Battery Top Spacer_v2 (Autodesk Fusion 360 design; units mm, degrees)
Autodesk Fusion 360 part; units mm, degrees
sketch "Sketch1" plane through (0, 0, 0) normal (1, 0, 0) x (0, 1, 0)
  line L0 (7.1607, -3.9) -> (12.8393, -3.9)
  line L1 (4.5, -8.2) -> (4.5, -6.5607)
  line L2 (12.8393, 3.9) -> (7.1607, 3.9)
  arc A0 (6.8786, -8.5414) -> (6.7372, -8.2) centre (6.7372, -8.4) ccw
  circle A1 centre (10, 0) radius 2.1
  arc A2 (5.1, -10) -> (5.5978, -9.8222) centre (5.1591, -9.3798) ccw
  line L3 (12.8393, 3.9) -> (7.1607, 3.9)
  line L4 (6.1, 2.8393) -> (6.1, -2.8393)
  line L5 (6.7372, -8.2) -> (4.5, -8.2)
  line L6 (6.1, 2.8393) -> (6.1, -2.8393)
  line L7 (4.5, -6.5607) -> (7.1607, -3.9)
  line L8 (5.5978, -9.8222) -> (6.8786, -8.5414)
  arc A3 (5.1, -10) -> (5.5978, -9.8222) centre (5.1591, -9.3798) ccw
  arc A4 (6.8786, -8.5414) -> (6.7372, -8.2) centre (6.7372, -8.4) ccw
  line L9 (6.7372, -8.2) -> (4.5, -8.2)
  line L10 (4.5, -8.2) -> (4.5, -6.5607)
  line L11 (4.5, -6.5607) -> (7.1607, -3.9)
  line L12 (5.5978, -9.8222) -> (6.8786, -8.5414)
  line L13 (7.1607, -3.9) -> (12.8393, -3.9)
  arc A5 (14.4022, -9.8222) -> (14.9, -10) centre (14.8416, -9.3778) ccw
  line L14 (26.7372, -8.2) -> (24.5, -8.2)
  line L15 (-18.2, 3.2628) -> (-18.2, 5.5)
  line L16 (33.2628, 8.2) -> (35.5, 8.2)
  line L17 (-18.2, 3.2628) -> (-18.2, 5.5)
  line L18 (24.5, -6.5607) -> (27.1607, -3.9)
  arc A6 (-14.8314, -10) -> (-14.4022, -9.8222) centre (-14.8314, -9.3929) ccw
  arc A7 (26.8786, -8.5414) -> (26.7372, -8.2) centre (26.7372, -8.4) ccw
  line L19 (38.2, 5.5) -> (38.2, 3.2628)
  arc A8 (38.2, 3.2628) -> (38.5414, 3.1214) centre (38.4, 3.2628) ccw
  line L20 (13.1214, -8.5414) -> (14.4022, -9.8222)
  arc A9 (40, 9.5) -> (39.5, 10) centre (39.5, 9.5) ccw
  arc A10 (-13.1214, -8.5414) -> (-13.2628, -8.2) centre (-13.2628, -8.4) ccw
  line L21 (22.7, -8.2) -> (17.3, -8.2)
  line L22 (36.5607, -5.5) -> (33.9, -2.8393)
  line L23 (-20, -4.8314) -> (-20, -9.5)
  line L24 (36.5607, 5.5) -> (38.2, 5.5)
  arc A11 (-18.2, -3.2628) -> (-18.5414, -3.1214) centre (-18.4, -3.2628) ccw
  arc A12 (39.5, -10) -> (40, -9.5) centre (39.5, -9.5) ccw
  arc A13 (33.1214, 8.5414) -> (33.2628, 8.2) centre (33.2628, 8.4) ccw
  line L25 (33.2628, 8.2) -> (35.5, 8.2)
  arc A14 (-14.8314, -10) -> (-14.4022, -9.8222) centre (-14.8314, -9.3929) ccw
  line L26 (40, -9.5) -> (40, -4.8314)
  line L27 (-13.2628, -8.2) -> (-15.5, -8.2)
  line L28 (38.2, 5.5) -> (38.2, 3.2628)
  line L29 (-13.2628, -8.2) -> (-15.5, -8.2)
  line L30 (33.9, 2.8393) -> (36.5607, 5.5)
  line L31 (33.1214, -8.5414) -> (34.4022, -9.8222)
  line L32 (-18.2, 5.5) -> (-16.5607, 5.5)
  line L33 (39.8222, -4.4022) -> (38.5414, -3.1214)
  arc A15 (34.4022, -9.8222) -> (34.8314, -10) centre (34.8314, -9.3929) ccw
  arc A16 (38.5414, -3.1214) -> (38.2, -3.2628) centre (38.4, -3.2628) ccw
  line L34 (35.5, -8.2) -> (33.2628, -8.2)
  line L35 (15.5, -6.5607) -> (15.5, -8.2)
  line L36 (-14.9, 10) -> (-19.5, 10)
  line L37 (32.8393, -3.9) -> (35.5, -6.5607)
  arc A17 (25.1, -10) -> (25.5978, -9.8222) centre (25.1584, -9.3778) ccw
  line L38 (24.5, -6.5607) -> (27.1607, -3.9)
  line L39 (15.5, -6.5607) -> (15.5, -8.2)
  line L40 (39.8222, -4.4022) -> (38.5414, -3.1214)
  line L41 (36.5607, -5.5) -> (33.9, -2.8393)
  arc A18 (38.5414, -3.1214) -> (38.2, -3.2628) centre (38.4, -3.2628) ccw
  arc A19 (26.8786, -8.5414) -> (26.7372, -8.2) centre (26.7372, -8.4) ccw
  arc A20 (13.2628, -8.2) -> (13.1214, -8.5414) centre (13.2628, -8.4) ccw
  line L42 (34.8314, -10) -> (39.5, -10)
  line L43 (-14.4022, -9.8222) -> (-13.1214, -8.5414)
  line L44 (26.1, -2.8393) -> (22.7, -6.2393)
  line L45 (38.2, -5.5) -> (36.5607, -5.5)
  line L46 (22.7, -6.2393) -> (22.7, -8.2)
  line L47 (35.5, -6.5607) -> (35.5, -8.2)
  arc A21 (-13.1214, -8.5414) -> (-13.2628, -8.2) centre (-13.2628, -8.4) ccw
  line L48 (24.5, -8.2) -> (24.5, -6.5607)
  line L49 (36.5607, 5.5) -> (38.2, 5.5)
  line L50 (35.5, -6.5607) -> (35.5, -8.2)
  arc A22 (33.1214, 8.5414) -> (33.2628, 8.2) centre (33.2628, 8.4) ccw
  arc A23 (-14.4022, 9.8222) -> (-14.9, 10) centre (-14.8416, 9.3778) ccw
  arc A24 (33.2628, -8.2) -> (33.1214, -8.5414) centre (33.2628, -8.4) ccw
  arc A25 (39.5, -10) -> (40, -9.5) centre (39.5, -9.5) ccw
  line L51 (24.5, -8.2) -> (24.5, -6.5607)
  line L52 (34.8314, -10) -> (39.5, -10)
  line L53 (38.2, -3.2628) -> (38.2, -5.5)
  line L54 (22.7, -6.2393) -> (22.7, -8.2)
  line L55 (40, -9.5) -> (40, -4.8314)
  line L56 (26.7372, -8.2) -> (24.5, -8.2)
  line L57 (25.5978, -9.8222) -> (26.8786, -8.5414)
  line L58 (17.3, -6.2393) -> (13.9, -2.8393)
  line L59 (14.9, -10) -> (25.1, -10)
  line L60 (15.5, -8.2) -> (13.2628, -8.2)
  line L61 (25.5978, -9.8222) -> (26.8786, -8.5414)
  arc A26 (25.1, -10) -> (25.5978, -9.8222) centre (25.1584, -9.3778) ccw
  line L62 (13.1214, -8.5414) -> (14.4022, -9.8222)
  line L63 (12.8393, -3.9) -> (15.5, -6.5607)
  line L64 (12.8393, -3.9) -> (15.5, -6.5607)
  arc A27 (13.2628, -8.2) -> (13.1214, -8.5414) centre (13.2628, -8.4) ccw
  line L65 (22.7, -8.2) -> (17.3, -8.2)
  line L66 (17.3, -8.2) -> (17.3, -6.2393)
  line L67 (26.1, -2.8393) -> (22.7, -6.2393)
  line L68 (14.9, -10) -> (25.1, -10)
  line L69 (17.3, -6.2393) -> (13.9, -2.8393)
  arc A28 (14.4022, -9.8222) -> (14.9, -10) centre (14.8416, -9.3778) ccw
  line L70 (17.3, -8.2) -> (17.3, -6.2393)
  line L71 (15.5, -8.2) -> (13.2628, -8.2)
  arc A29 (-18.5414, 3.1214) -> (-18.2, 3.2628) centre (-18.4, 3.2628) ccw
  arc A30 (-20, -9.5) -> (-19.5, -10) centre (-19.5, -9.5) ccw
  arc A31 (39.8222, 4.4022) -> (40, 4.8314) centre (39.3929, 4.8314) ccw
  line L72 (-13.9, -2.8393) -> (-16.5607, -5.5)
  arc A32 (-18.2, -3.2628) -> (-18.5414, -3.1214) centre (-18.4, -3.2628) ccw
  line L73 (24.5, 8.2) -> (26.7372, 8.2)
  line L74 (35.5, 8.2) -> (35.5, 6.5607)
  line L75 (26.1, 2.8393) -> (26.1, -2.8393)
  line L76 (-18.2, -5.5) -> (-18.2, -3.2628)
  arc A33 (39.8222, 4.4022) -> (40, 4.8314) centre (39.3929, 4.8314) ccw
  line L77 (-20, 9.5) -> (-20, 4.8314)
  line L78 (13.2628, 8.2) -> (15.5, 8.2)
  line L79 (17.3, 8.2) -> (22.7, 8.2)
  line L80 (-15.5, -6.5607) -> (-12.8393, -3.9)
  line L81 (-19.8222, 4.4022) -> (-18.5414, 3.1214)
  arc A34 (-19.8222, -4.4022) -> (-20, -4.8314) centre (-19.3929, -4.8314) ccw
  arc A35 (38.2, 3.2628) -> (38.5414, 3.1214) centre (38.4, 3.2628) ccw
  line L82 (15.5, 8.2) -> (15.5, 6.5607)
  arc A36 (-20, 4.8314) -> (-19.8222, 4.4022) centre (-19.3929, 4.8314) ccw
  line L83 (25.1, 10) -> (14.9, 10)
  line L84 (-15.5, 6.5607) -> (-15.5, 8.2)
  line L85 (26.1, 2.8393) -> (26.1, -2.8393)
  arc A37 (-20, 4.8314) -> (-19.8222, 4.4022) centre (-19.3929, 4.8314) ccw
  arc A38 (-20, -9.5) -> (-19.5, -10) centre (-19.5, -9.5) ccw
  line L86 (-12.8393, 3.9) -> (-15.5, 6.5607)
  line L87 (17.3, 8.2) -> (22.7, 8.2)
  arc A39 (14.9, 10) -> (14.4022, 9.8222) centre (14.8416, 9.3778) ccw
  line L88 (33.9, -2.8393) -> (33.9, 2.8393)
  line L89 (33.9, -2.8393) -> (33.9, 2.8393)
  line L90 (13.9, 2.8393) -> (17.3, 6.2393)
  line L91 (33.9, 2.8393) -> (36.5607, 5.5)
  line L92 (-13.1214, 8.5414) -> (-14.4022, 9.8222)
  line L93 (25.1, 10) -> (14.9, 10)
  line L94 (-15.5, 8.2) -> (-13.2628, 8.2)
  arc A40 (14.9, 10) -> (14.4022, 9.8222) centre (14.8416, 9.3778) ccw
  line L95 (17.3, 6.2393) -> (17.3, 8.2)
  line L96 (15.5, 6.5607) -> (12.8393, 3.9)
  line L97 (-15.5, 6.5607) -> (-15.5, 8.2)
  line L98 (39.5, 10) -> (34.9, 10)
  arc A41 (25.5978, 9.8222) -> (25.1, 10) centre (25.1584, 9.3778) ccw
  arc A42 (34.9, 10) -> (34.4022, 9.8222) centre (34.8416, 9.3778) ccw
  arc A43 (-13.2628, 8.2) -> (-13.1214, 8.5414) centre (-13.2628, 8.4) ccw
  line L99 (13.9, -2.8393) -> (13.9, 2.8393)
  line L100 (15.5, 8.2) -> (15.5, 6.5607)
  line L101 (-18.5414, -3.1214) -> (-19.8222, -4.4022)
  line L102 (-18.2, 5.5) -> (-16.5607, 5.5)
  line L103 (-19.5, -10) -> (-14.8314, -10)
  arc A44 (13.1214, 8.5414) -> (13.2628, 8.2) centre (13.2628, 8.4) ccw
  line L104 (-19.5, -10) -> (-14.8314, -10)
  line L105 (38.5414, 3.1214) -> (39.8222, 4.4022)
  arc A45 (-13.2628, 8.2) -> (-13.1214, 8.5414) centre (-13.2628, 8.4) ccw
  line L106 (-18.2, -5.5) -> (-18.2, -3.2628)
  arc A46 (33.2628, -8.2) -> (33.1214, -8.5414) centre (33.2628, -8.4) ccw
  arc A47 (40, -4.8314) -> (39.8222, -4.4022) centre (39.3929, -4.8314) ccw
  line L107 (-18.5414, -3.1214) -> (-19.8222, -4.4022)
  line L108 (-16.5607, 5.5) -> (-13.9, 2.8393)
  line L109 (-20, -4.8314) -> (-20, -9.5)
  line L110 (14.4022, 9.8222) -> (13.1214, 8.5414)
  line L111 (-20, 9.5) -> (-20, 4.8314)
  line L112 (15.5, 6.5607) -> (12.8393, 3.9)
  line L113 (38.2, -3.2628) -> (38.2, -5.5)
  line L114 (-16.5607, -5.5) -> (-18.2, -5.5)
  line L115 (-14.4022, -9.8222) -> (-13.1214, -8.5414)
  line L116 (-12.8393, 3.9) -> (-15.5, 6.5607)
  line L117 (-13.1214, 8.5414) -> (-14.4022, 9.8222)
  line L118 (32.8393, -3.9) -> (35.5, -6.5607)
  line L119 (35.5, -8.2) -> (33.2628, -8.2)
  line L120 (35.5, 6.5607) -> (32.8393, 3.9)
  line L121 (26.8786, 8.5414) -> (25.5978, 9.8222)
  line L122 (17.3, 6.2393) -> (17.3, 8.2)
  arc A48 (-19.8222, -4.4022) -> (-20, -4.8314) centre (-19.3929, -4.8314) ccw
  line L123 (-16.5607, 5.5) -> (-13.9, 2.8393)
  arc A49 (13.1214, 8.5414) -> (13.2628, 8.2) centre (13.2628, 8.4) ccw
  arc A50 (34.9, 10) -> (34.4022, 9.8222) centre (34.8416, 9.3778) ccw
  arc A51 (34.4022, -9.8222) -> (34.8314, -10) centre (34.8314, -9.3929) ccw
  line L124 (-14.9, 10) -> (-19.5, 10)
  line L125 (22.7, 8.2) -> (22.7, 6.2393)
  arc A52 (26.7372, 8.2) -> (26.8786, 8.5414) centre (26.7372, 8.4) ccw
  line L126 (27.1607, 3.9) -> (24.5, 6.5607)
  line L127 (38.5414, 3.1214) -> (39.8222, 4.4022)
  line L128 (34.4022, 9.8222) -> (33.1214, 8.5414)
  line L129 (40, 4.8314) -> (40, 9.5)
  line L130 (35.5, 6.5607) -> (32.8393, 3.9)
  line L131 (39.5, 10) -> (34.9, 10)
  line L132 (-15.5, -8.2) -> (-15.5, -6.5607)
  line L133 (35.5, 8.2) -> (35.5, 6.5607)
  line L134 (38.2, -5.5) -> (36.5607, -5.5)
  line L135 (-15.5, 8.2) -> (-13.2628, 8.2)
  line L136 (-15.5, -6.5607) -> (-12.8393, -3.9)
  line L137 (34.4022, 9.8222) -> (33.1214, 8.5414)
  arc A53 (-19.5, 10) -> (-20, 9.5) centre (-19.5, 9.5) ccw
  arc A54 (-19.5, 10) -> (-20, 9.5) centre (-19.5, 9.5) ccw
  line L138 (40, 4.8314) -> (40, 9.5)
  arc A55 (40, 9.5) -> (39.5, 10) centre (39.5, 9.5) ccw
  line L139 (27.1607, 3.9) -> (24.5, 6.5607)
  arc A56 (26.7372, 8.2) -> (26.8786, 8.5414) centre (26.7372, 8.4) ccw
  line L140 (-16.5607, -5.5) -> (-18.2, -5.5)
  line L141 (-19.8222, 4.4022) -> (-18.5414, 3.1214)
  arc A57 (40, -4.8314) -> (39.8222, -4.4022) centre (39.3929, -4.8314) ccw
  line L142 (-13.9, -2.8393) -> (-16.5607, -5.5)
  line L143 (-15.5, -8.2) -> (-15.5, -6.5607)
  arc A58 (-14.4022, 9.8222) -> (-14.9, 10) centre (-14.8416, 9.3778) ccw
  line L144 (33.1214, -8.5414) -> (34.4022, -9.8222)
  arc A59 (-18.5414, 3.1214) -> (-18.2, 3.2628) centre (-18.4, 3.2628) ccw
  line L145 (2.7, 8.2) -> (2.7, 6.2393)
  line L146 (-5.5978, 9.8222) -> (-6.8786, 8.5414)
  line L147 (-4.5, 8.2) -> (-4.5, 6.5607)
  arc A60 (-6.8786, 8.5414) -> (-6.7372, 8.2) centre (-6.7372, 8.4) ccw
  arc A61 (-5.1, 10) -> (-5.5978, 9.8222) centre (-5.1584, 9.3778) ccw
  line L148 (-2.7, 6.2393) -> (-2.7, 8.2)
  line L149 (-6.7372, 8.2) -> (-4.5, 8.2)
  line L150 (4.5, 6.5607) -> (4.5, 8.2)
  line L151 (-5.5978, 9.8222) -> (-6.8786, 8.5414)
  line L152 (7.1607, 3.9) -> (4.5, 6.5607)
  line L153 (6.8786, 8.5414) -> (5.5978, 9.8222)
  line L154 (2.7, 8.2) -> (2.7, 6.2393)
  line L155 (7.1607, 3.9) -> (4.5, 6.5607)
  arc A62 (-5.1, 10) -> (-5.5978, 9.8222) centre (-5.1584, 9.3778) ccw
  line L156 (-5.1, -10) -> (5.1, -10)
  arc A63 (5.5978, 9.8222) -> (5.1, 10) centre (5.1584, 9.3778) ccw
  line L157 (-4.5, 6.5607) -> (-7.1607, 3.9)
  line L158 (-2.7, 8.2) -> (2.7, 8.2)
  line L159 (32.8393, 3.9) -> (27.1607, 3.9)
  line L160 (5.1, 10) -> (-5.1, 10)
  circle A64 centre (30, 0) radius 2.1
  line L161 (5.1, 10) -> (-5.1, 10)
  arc A65 (6.7372, 8.2) -> (6.8786, 8.5414) centre (6.7372, 8.4) ccw
  arc A66 (5.5978, 9.8222) -> (5.1, 10) centre (5.1584, 9.3778) ccw
  line L162 (-4.5, 8.2) -> (-4.5, 6.5607)
  line L163 (4.5, 6.5607) -> (4.5, 8.2)
  arc A67 (6.7372, 8.2) -> (6.8786, 8.5414) centre (6.7372, 8.4) ccw
  line L164 (6.8786, 8.5414) -> (5.5978, 9.8222)
  line L165 (-4.5, 6.5607) -> (-7.1607, 3.9)
  arc A68 (-6.8786, 8.5414) -> (-6.7372, 8.2) centre (-6.7372, 8.4) ccw
  line L166 (-2.7, 6.2393) -> (-2.7, 8.2)
  line L167 (-7.1607, 3.9) -> (-12.8393, 3.9)
  line L168 (4.5, 8.2) -> (6.7372, 8.2)
  line L169 (4.5, 8.2) -> (6.7372, 8.2)
  line L170 (27.1607, -3.9) -> (32.8393, -3.9)
  line L171 (32.8393, 3.9) -> (27.1607, 3.9)
  line L172 (24.5, 6.5607) -> (24.5, 8.2)
  line L173 (13.2628, 8.2) -> (15.5, 8.2)
  line L174 (27.1607, -3.9) -> (32.8393, -3.9)
  line L175 (-13.9, 2.8393) -> (-13.9, -2.8393)
  arc A69 (25.5978, 9.8222) -> (25.1, 10) centre (25.1584, 9.3778) ccw
  line L176 (13.9, -2.8393) -> (13.9, 2.8393)
  line L177 (-6.1, 2.8393) -> (-2.7, 6.2393)
  line L178 (-2.7, 8.2) -> (2.7, 8.2)
  line L179 (22.7, 6.2393) -> (26.1, 2.8393)
  line L180 (2.7, 6.2393) -> (6.1, 2.8393)
  line L181 (2.7, 6.2393) -> (6.1, 2.8393)
  line L182 (-6.7372, 8.2) -> (-4.5, 8.2)
  circle A70 centre (-10, 0) radius 2.1
  line L183 (22.7, 8.2) -> (22.7, 6.2393)
  line L184 (-13.9, 2.8393) -> (-13.9, -2.8393)
  line L185 (24.5, 6.5607) -> (24.5, 8.2)
  line L186 (24.5, 8.2) -> (26.7372, 8.2)
  line L187 (22.7, 6.2393) -> (26.1, 2.8393)
  line L188 (-12.8393, -3.9) -> (-7.1607, -3.9)
  line L189 (-6.1, 2.8393) -> (-2.7, 6.2393)
  line L190 (13.9, 2.8393) -> (17.3, 6.2393)
  line L191 (26.8786, 8.5414) -> (25.5978, 9.8222)
  line L192 (-12.8393, -3.9) -> (-7.1607, -3.9)
  line L193 (-7.1607, 3.9) -> (-12.8393, 3.9)
  line L194 (14.4022, 9.8222) -> (13.1214, 8.5414)
  arc A71 (-6.7372, -8.2) -> (-6.8786, -8.5414) centre (-6.7372, -8.4) ccw
  line L195 (-6.8786, -8.5414) -> (-5.5978, -9.8222)
  line L196 (-2.7, -8.2) -> (-2.7, -6.2393)
  line L197 (-6.8786, -8.5414) -> (-5.5978, -9.8222)
  line L198 (2.7, -6.2393) -> (2.7, -8.2)
  arc A72 (-5.5978, -9.8222) -> (-5.1, -10) centre (-5.1591, -9.3798) ccw
  line L199 (2.7, -8.2) -> (-2.7, -8.2)
  arc A73 (-6.7372, -8.2) -> (-6.8786, -8.5414) centre (-6.7372, -8.4) ccw
  line L200 (2.7, -6.2393) -> (2.7, -8.2)
  line L201 (-4.5, -6.5607) -> (-4.5, -8.2)
  line L202 (-2.7, -6.2393) -> (-6.1, -2.8393)
  line L203 (-7.1607, -3.9) -> (-4.5, -6.5607)
  line L204 (-4.5, -6.5607) -> (-4.5, -8.2)
  line L205 (-2.7, -8.2) -> (-2.7, -6.2393)
  line L206 (-7.1607, -3.9) -> (-4.5, -6.5607)
  line L207 (-4.5, -8.2) -> (-6.7372, -8.2)
  arc A74 (-5.5978, -9.8222) -> (-5.1, -10) centre (-5.1591, -9.3798) ccw
  line L208 (-5.1, -10) -> (5.1, -10)
  line L209 (-6.1, -2.8393) -> (-6.1, 2.8393)
  line L210 (-4.5, -8.2) -> (-6.7372, -8.2)
  line L211 (2.7, -8.2) -> (-2.7, -8.2)
  line L212 (-2.7, -6.2393) -> (-6.1, -2.8393)
  line L213 (6.1, -2.8393) -> (2.7, -6.2393)
  line L214 (6.1, -2.8393) -> (2.7, -6.2393)
  line L215 (-6.1, -2.8393) -> (-6.1, 2.8393)
  line L216 (-4.6, -6.6021) -> (-4.6, -8.1)
  line L217 (-4.6, -8.1) -> (-6.7372, -8.1)
  arc A75 (-6.7372, -8.1) -> (-6.9493, -8.6121) centre (-6.7372, -8.4) ccw
  line L218 (-6.9493, -8.6121) -> (-5.6692, -9.8922)
  arc A76 (-5.6692, -9.8922) -> (-5.0954, -10.1) centre (-5.1591, -9.3798) ccw
  line L219 (-5.0954, -10.1) -> (5.0954, -10.1)
  arc A77 (5.0954, -10.1) -> (5.6692, -9.8922) centre (5.1591, -9.3798) ccw
  line L220 (5.6692, -9.8922) -> (6.9493, -8.6121)
  arc A78 (6.9493, -8.6121) -> (6.7372, -8.1) centre (6.7372, -8.4) ccw
  line L221 (6.7372, -8.1) -> (4.6, -8.1)
  line L222 (4.6, -8.1) -> (4.6, -6.6021)
  line L223 (4.6, -6.6021) -> (7.2021, -4)
  line L224 (7.2021, -4) -> (12.7979, -4)
  line L225 (12.7979, -4) -> (15.4, -6.6021)
  line L226 (15.4, -6.6021) -> (15.4, -8.1)
  line L227 (15.4, -8.1) -> (13.2628, -8.1)
  arc A79 (13.2628, -8.1) -> (13.0507, -8.6121) centre (13.2628, -8.4) ccw
  line L228 (13.0507, -8.6121) -> (14.3305, -9.892)
  arc A80 (14.3305, -9.892) -> (14.9045, -10.1) centre (14.8416, -9.3778) ccw
  line L229 (14.9045, -10.1) -> (25.0955, -10.1)
  arc A81 (25.0955, -10.1) -> (25.6695, -9.892) centre (25.1584, -9.3778) ccw
  line L230 (25.6695, -9.892) -> (26.9493, -8.6121)
  arc A82 (26.9493, -8.6121) -> (26.7372, -8.1) centre (26.7372, -8.4) ccw
  line L231 (26.7372, -8.1) -> (24.6, -8.1)
  line L232 (24.6, -8.1) -> (24.6, -6.6021)
  line L233 (24.6, -6.6021) -> (27.2021, -4)
  line L234 (27.2021, -4) -> (32.7979, -4)
  line L235 (32.7979, -4) -> (35.4, -6.6021)
  line L236 (35.4, -6.6021) -> (35.4, -8.1)
  line L237 (35.4, -8.1) -> (33.2628, -8.1)
  arc A83 (33.2628, -8.1) -> (33.0507, -8.6121) centre (33.2628, -8.4) ccw
  line L238 (33.0507, -8.6121) -> (34.3315, -9.8929)
  arc A84 (34.3315, -9.8929) -> (34.8314, -10.1) centre (34.8314, -9.3929) ccw
  line L239 (34.8314, -10.1) -> (39.5, -10.1)
  arc A85 (39.5, -10.1) -> (40.1, -9.5) centre (39.5, -9.5) ccw
  line L240 (40.1, -9.5) -> (40.1, -4.8314)
  arc A86 (40.1, -4.8314) -> (39.8929, -4.3315) centre (39.3929, -4.8314) ccw
  line L241 (39.8929, -4.3315) -> (38.6121, -3.0507)
  arc A87 (38.6121, -3.0507) -> (38.1, -3.2628) centre (38.4, -3.2628) ccw
  line L242 (38.1, -3.2628) -> (38.1, -5.4)
  line L243 (38.1, -5.4) -> (36.6021, -5.4)
  line L244 (36.6021, -5.4) -> (34, -2.7979)
  line L245 (34, -2.7979) -> (34, 2.7979)
  line L246 (34, 2.7979) -> (36.6021, 5.4)
  line L247 (36.6021, 5.4) -> (38.1, 5.4)
  line L248 (38.1, 5.4) -> (38.1, 3.2628)
  arc A88 (38.1, 3.2628) -> (38.6121, 3.0507) centre (38.4, 3.2628) ccw
  line L249 (38.6121, 3.0507) -> (39.8929, 4.3315)
  arc A89 (39.8929, 4.3315) -> (40.1, 4.8314) centre (39.3929, 4.8314) ccw
  line L250 (40.1, 4.8314) -> (40.1, 9.5)
  arc A90 (40.1, 9.5) -> (39.5, 10.1) centre (39.5, 9.5) ccw
  line L251 (39.5, 10.1) -> (34.9045, 10.1)
  arc A91 (34.9045, 10.1) -> (34.3305, 9.892) centre (34.8416, 9.3778) ccw
  line L252 (34.3305, 9.892) -> (33.0507, 8.6121)
  arc A92 (33.0507, 8.6121) -> (33.2628, 8.1) centre (33.2628, 8.4) ccw
  line L253 (33.2628, 8.1) -> (35.4, 8.1)
  line L254 (35.4, 8.1) -> (35.4, 6.6021)
  line L255 (35.4, 6.6021) -> (32.7979, 4)
  line L256 (32.7979, 4) -> (27.2021, 4)
  line L257 (27.2021, 4) -> (24.6, 6.6021)
  line L258 (24.6, 6.6021) -> (24.6, 8.1)
  line L259 (24.6, 8.1) -> (26.7372, 8.1)
  arc A93 (26.7372, 8.1) -> (26.9493, 8.6121) centre (26.7372, 8.4) ccw
  line L260 (26.9493, 8.6121) -> (25.6695, 9.892)
  arc A94 (25.6695, 9.892) -> (25.0955, 10.1) centre (25.1584, 9.3778) ccw
  line L261 (25.0955, 10.1) -> (14.9045, 10.1)
  arc A95 (14.9045, 10.1) -> (14.3274, 9.8888) centre (14.8416, 9.3778) ccw
  line L262 (14.3274, 9.8888) -> (13.0507, 8.6121)
  arc A96 (13.0507, 8.6121) -> (13.2628, 8.1) centre (13.2628, 8.4) ccw
  line L263 (13.2628, 8.1) -> (15.4, 8.1)
  line L264 (15.4, 8.1) -> (15.4, 6.6021)
  line L265 (15.4, 6.6021) -> (12.7979, 4)
  line L266 (12.7979, 4) -> (7.2021, 4)
  line L267 (7.2021, 4) -> (4.6, 6.6021)
  line L268 (4.6, 6.6021) -> (4.6, 8.1)
  line L269 (4.6, 8.1) -> (6.7372, 8.1)
  arc A97 (6.7372, 8.1) -> (6.9493, 8.6121) centre (6.7372, 8.4) ccw
  line L270 (6.9493, 8.6121) -> (5.6695, 9.892)
  arc A98 (5.6695, 9.892) -> (5.0955, 10.1) centre (5.1584, 9.3778) ccw
  line L271 (5.0955, 10.1) -> (-5.0955, 10.1)
  arc A99 (-5.0955, 10.1) -> (-5.6695, 9.892) centre (-5.1584, 9.3778) ccw
  line L272 (-5.6695, 9.892) -> (-6.9493, 8.6121)
  arc A100 (-6.9493, 8.6121) -> (-6.7372, 8.1) centre (-6.7372, 8.4) ccw
  line L273 (-6.7372, 8.1) -> (-4.6, 8.1)
  line L274 (-4.6, 8.1) -> (-4.6, 6.6021)
  line L275 (-4.6, 6.6021) -> (-7.2021, 4)
  line L276 (-7.2021, 4) -> (-12.7979, 4)
  line L277 (-12.7979, 4) -> (-15.4, 6.6021)
  line L278 (-15.4, 6.6021) -> (-15.4, 8.1)
  line L279 (-15.4, 8.1) -> (-13.2628, 8.1)
  arc A101 (-13.2628, 8.1) -> (-13.0507, 8.6121) centre (-13.2628, 8.4) ccw
  line L280 (-13.0507, 8.6121) -> (-14.3305, 9.892)
  arc A102 (-14.3305, 9.892) -> (-14.9045, 10.1) centre (-14.8416, 9.3778) ccw
  line L281 (-14.9045, 10.1) -> (-19.5, 10.1)
  arc A103 (-19.5, 10.1) -> (-20.1, 9.5) centre (-19.5, 9.5) ccw
  line L282 (-20.1, 9.5) -> (-20.1, 4.8314)
  arc A104 (-20.1, 4.8314) -> (-19.8929, 4.3315) centre (-19.3929, 4.8314) ccw
  line L283 (-19.8929, 4.3315) -> (-18.6121, 3.0507)
  arc A105 (-18.6121, 3.0507) -> (-18.1, 3.2628) centre (-18.4, 3.2628) ccw
  line L284 (-18.1, 3.2628) -> (-18.1, 5.4)
  line L285 (-18.1, 5.4) -> (-16.6021, 5.4)
  line L286 (-16.6021, 5.4) -> (-14, 2.7979)
  line L287 (-14, 2.7979) -> (-14, -2.7979)
  line L288 (-14, -2.7979) -> (-16.6021, -5.4)
  line L289 (-16.6021, -5.4) -> (-18.1, -5.4)
  line L290 (-18.1, -5.4) -> (-18.1, -3.2628)
  arc A106 (-18.1, -3.2628) -> (-18.6121, -3.0507) centre (-18.4, -3.2628) ccw
  line L291 (-18.6121, -3.0507) -> (-19.8929, -4.3315)
  arc A107 (-19.8929, -4.3315) -> (-20.1, -4.8314) centre (-19.3929, -4.8314) ccw
  line L292 (-20.1, -4.8314) -> (-20.1, -9.5)
  arc A108 (-20.1, -9.5) -> (-19.5, -10.1) centre (-19.5, -9.5) ccw
  line L293 (-19.5, -10.1) -> (-14.8314, -10.1)
  arc A109 (-14.8314, -10.1) -> (-14.3315, -9.8929) centre (-14.8314, -9.3929) ccw
  line L294 (-14.3315, -9.8929) -> (-13.0507, -8.6121)
  arc A110 (-13.0507, -8.6121) -> (-13.2628, -8.1) centre (-13.2628, -8.4) ccw
  line L295 (-13.2628, -8.1) -> (-15.4, -8.1)
  line L296 (-15.4, -8.1) -> (-15.4, -6.6021)
  line L297 (-15.4, -6.6021) -> (-12.7979, -4)
  line L298 (-12.7979, -4) -> (-7.2021, -4)
  line L299 (-7.2021, -4) -> (-4.6, -6.6021)
  line L300 (19.5, -10) -> (19.5, -20)
  line L301 (19.5, -20) -> (-19.5, -20)
  line L302 (-19.5, -20) -> (-19.5, -10)
  line L303 (-19.5, -10) -> (-14.4689, -10)
  line L304 (-5.5308, -10) -> (5.5308, -10)
  line L305 (14.4696, -10) -> (19.5, -10)
  point P0 (30, 0)
  point P1 (10, 0)
  point P2 (-10, 0)
  point P3 (10, 0)
  dimension "d1" = 4.2
  dimension "d2" = 4.2
  dimension "d3" = 4.2
  dimension "d4" = 0.1
  dimension "d5" = 10
  constraint coincident P0 A64.centre
  constraint coincident P3 P1
  constraint coincident P2 A70.centre
  constraint horizontal L303
  constraint vertical L300
  constraint horizontal L301
  constraint vertical L302
  constraint coincident A109 L303.end
  constraint coincident A76 L304.start
  constraint collinear L303 L304
  constraint coincident A77 L304.end
  constraint coincident A80 L305.start
  constraint collinear L304 L305
  measures "d1" diameter of A64
  measures "d2" diameter of A1
  measures "d3" diameter of A70
  measures "d5" distance of A30.end L301.end
extrude "Extrude1" add sketch "Sketch1" along normal blind 70 contours L216 L217 A75 L218 A76 L219 A77 L220 A78 L221 L222 L223 L224 L225 L226 L227 A79 L228 A80 L229 L293 A109 L294 A110 L295 L296 L297 L298 L299 L300 L301 L302
